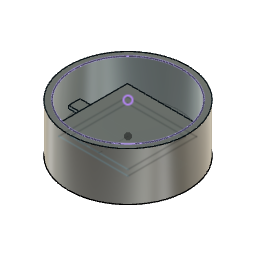
Charger v1 (Autodesk Fusion 360 design; units mm, degrees)
Autodesk Fusion 360 part; units mm, degrees
note: some values were not read from the file. Set by a fixed rule: which sketch regions a step uses.
sketch "Sketch1" plane through (0, 0, 0) normal (0, 0, 1) x (1, 0, 0)
  circle A0 centre (0, 0) radius 7.925
  circle A1 centre (0, 0) radius 8.925
  dimension "d1" = 15.85
  dimension "d4" = 1
  constraint coincident A0.centre A1.centre
  measures "d1" diameter of A0
extrude "Extrude1" add sketch "Sketch1" along normal blind 1 contours A0 | A1 makes body 1
sketch "Sketch2" plane through (0, 0, 1) normal (0, 0, 1) x (-1, 0, 0)
  circle A0 centre (0, 0) radius 8.925
  circle A1 centre (0, 0) radius 7.925
  circle A2 centre (0, 0) radius 1.225
  dimension "d5" = 2.45
  constraint concentric A1 A2
  measures "d5" diameter of A2
extrude "Extrude2" add sketch "Sketch2" along normal blind 1.5 bodies 1
sketch "Sketch1 (2)" plane through (0, 0, 0) normal (0, 0, -1) x (1, 0, 0) in component "Charger Bottom"
  circle A0 centre (0, 0) radius 8.925
  circle A1 centre (0, 0) radius 8.925
  circle A2 centre (0, 0) radius 9.425
  circle A3 centre (0, 0) radius 10.425
  dimension "d8" = 0.5
  dimension "d9" = 1.5
extrude "Extrude1'" add sketch "Sketch1 (2)" against normal blind 2.5 separate body contours A3 makes body 2 in component "Charger Bottom"
extrude "Extrude2'" add 1 faces at (10.0178, 0.9862, 2.5) along direction (0, 0, 1) blind 3 on bodies 2 bodies 2 in component "Charger Bottom"
sketch "Sketch2 (2)" plane through (0, 0, 2.5) normal (0, 0, 1) x (-1, 0, 0) in component "Charger Bottom"
  circle A0 centre (0, 0) radius 7.925
  circle A1 centre (0, 0) radius 8.925
  circle A2 centre (0, 0) radius 9.425
  circle A3 centre (0, 0) radius 10.425
  line L0 (10.425, 0.0113) -> (-10.425, 0.0113)
  line L1 (10.425, 1.0113) -> (-10.425, 1.0113)
  line L2 (10.425, -0.9887) -> (-10.425, -0.9887)
  dimension "d14" = 1
  dimension "d15" = -1
  constraint coincident A3 L0.start
  constraint coincident A3 L0.end
  constraint horizontal L0
extrude "Extrude3" add sketch "Sketch2 (2)" along normal blind 1 contours A0 L0 L2 | A0 A1 L0 L2 | A0 L0 L1 | A0 A1 L0 L1 | A1 A2 L0 L2 | A1 A2 L0 L1 | A0 A1 L0 L1 | A0 A1 L0 L2 | A1 A2 L0 L1 | A1 A2 L0 L2 bodies 2 in component "Charger Bottom"
extrude "Extrude4" cut 1 faces at (3.1235, 0.322, 2.5) along direction (0, 0, 1) blind 0.5 on bodies 2 bodies 2 in component "Charger Bottom"
sketch "Sketch3" plane through (0, 0, 3) normal (0, 0, -1) x (1, 0, 0) in component "Charger Bottom"
  arc A0 (-9.3706, 1.0113) -> (-9.373, -0.9887) centre (0, 0) ccw
  line L0 (-9.373, -0.9887) -> (9.373, -0.9887)
  arc A1 (9.373, -0.9887) -> (9.3706, 1.0113) centre (0, 0) ccw
  line L1 (9.3706, 1.0113) -> (-9.3706, 1.0113)
  line L2 (0, 0) -> (0, 5.05) construction
  line L3 (0, 5.05) -> (-5.05, 5.05) construction
  line L4 (-5.05, 5.05) -> (-5.05, -4.95)
  line L5 (-5.05, -4.95) -> (5.05, -4.95)
  line L6 (5.05, -4.95) -> (5.05, 5.05)
  line L7 (5.05, 5.05) -> (-5.05, 5.05)
  line L8 (6.05, 6.05) -> (-6.05, 6.05)
  line L9 (-6.05, 6.05) -> (-6.05, -5.95)
  line L10 (-6.05, -5.95) -> (6.05, -5.95)
  line L11 (6.05, -5.95) -> (6.05, 6.05)
  dimension "d20" = 5.05
  dimension "d21" = 5.05
  dimension "d22" = 10
  dimension "d23" = 10.1
  dimension "d24" = 1
  constraint coincident A0.centre A1.centre
  constraint perpendicular L1 L2
  constraint perpendicular L2 L3
  constraint perpendicular L3 L4
  constraint perpendicular L4 L5
  constraint perpendicular L5 L6
  measures "d20" distance of A0.centre L2.end
  measures "d21" distance of L2.end L3.end
  measures "d22" distance of L3.end L4.end
  measures "d23" distance of L4.end L5.end
extrude "Extrude6" add sketch "Sketch3" against normal blind 1 contours L1 L4 L6 L7 L8 L9 L11 | L0 L1 L4 L9 | L0 L4 L5 L6 L9 L10 L11 | L0 L1 L6 L11 bodies 2 in component "Charger Bottom"
extrude "Extrude5" cut sketch "Sketch3" against normal blind 0.5 contours L1 L4 L6 L7 | L0 L1 L4 L6 | L0 L4 L5 L6 bodies 2 in component "Charger Bottom"
sketch "Sketch4" plane through (0, 0, 4) normal (0, 0, 1) x (-1, 0, 0) in component "Charger Bottom"
  line L0 (-5.05, 5.05) -> (5.05, 5.05)
  line L1 (5.05, 5.05) -> (5.05, -4.95)
  line L2 (5.05, -4.95) -> (-5.05, -4.95)
  line L3 (-5.05, -4.95) -> (-5.05, 5.05)
  line L4 (-6.05, 6.05) -> (-6.05, -5.95)
  line L5 (-6.05, -5.95) -> (6.05, -5.95)
  line L6 (6.05, -5.95) -> (6.05, 6.05)
  line L7 (6.05, 6.05) -> (-6.05, 6.05)
  line L8 (5.05, -4.95) -> (-5.05, -4.95)
  line L9 (5.05, 5.05) -> (5.05, -4.95)
  line L10 (-5.05, 5.05) -> (5.05, 5.05)
  line L11 (-5.05, -4.95) -> (-5.05, 5.05)
extrude "Extrude7" add sketch "Sketch4" along normal blind 1 contours L0 L1 L2 L3 L8 L9 L10 L11 | L4 L5 L6 L7 bodies 2 in component "Charger Bottom"
extrude "Extrude8" add 1 faces at (10.0178, 0.9862, 5.5) along direction (0, 0, 1) blind 3 on bodies 2 bodies 2 in component "Charger Bottom"
sketch "Sketch5" plane through (0, 0, 8.5) normal (0, 0, 1) x (-1, 0, 0) in component "Charger Bottom"
  circle A0 centre (0, 0) radius 9.425
  circle A1 centre (0, 0) radius 10.425
  circle A2 centre (0, 0) radius 9.425
component "Charger Bottom" placed x (1, 0, 0) y (0, 1, 0) z (0, 0, 1) at (0, 0, 0)
equation "d1 = ( 31.7 / 2 ) * 1 mm"
equation "d5 = ( 4.9 / 2 ) * 1 mm"
